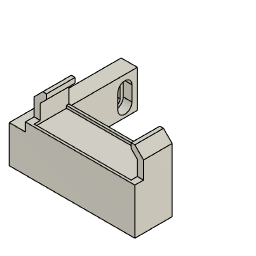
Nozzle brush (Autodesk Fusion 360 design; units mm, degrees)
Autodesk Fusion 360 part; units mm, degrees
sketch "Sketch1" plane through (0, 0, 0) normal (0, 1, 0) x (1, 0, 0)
  line L0 (0, 0) -> (6.5, 0)
  line L1 (6.5, 0) -> (6.5, -15)
  line L2 (6.5, -15) -> (0, -15)
  line L3 (0, -15) -> (0, 0)
  dimension "d1" = 6.5
  dimension "d2" = 15
  constraint horizontal L0
  constraint vertical L1
  constraint horizontal L2
  constraint vertical L3
  constraint coincident L0.start L3.end
  measures "d1" distance of L0.start L0.end
  measures "d2" distance of L0.start L2.end
extrude "Extrude1" add sketch "Sketch1" along normal blind 46.5
sketch "Sketch4" plane through (0, 0, 0) normal (0, -1, 0) x (1, 0, 0)
  line L0 (6.5, 15) -> (0, 15)
  line L1 (0, 15) -> (0, 0)
  line L2 (0, 0) -> (6.5, 0)
  line L3 (6.5, 0) -> (6.5, 15)
  line L4 (6.5, 15) -> (50.5, 15)
  line L5 (50.5, 15) -> (50.5, 29)
  line L6 (50.5, 29) -> (6.5, 29)
  line L7 (6.5, 29) -> (6.5, 15)
  line L8 (50.5, 15) -> (50.5, 0)
  line L9 (50.5, 0) -> (6.5, 0)
  dimension "d20" = 44
  dimension "d23" = 14
  dimension "d55" = 15
  constraint horizontal L4
  constraint vertical L5
  constraint horizontal L6
  constraint vertical L7
  constraint perpendicular L4 L8
  constraint coincident L2.end L3.start
  constraint horizontal L9
  constraint collinear L3 L7
  measures "d20" distance of L5.end L6.end
  measures "d23" distance of L4.end L5.end
  measures "d55" distance of L2 L4
extrude "Extrude5" add sketch "Sketch4" against normal blind 16.5
sketch "Sketch5" plane through (0, 16.5, 0) normal (0, 1, 0) x (-1, 0, 0)
  line L0 (-6.5, 15) -> (-6.5, 29)
  line L1 (-6.5, 29) -> (-50.5, 29)
  line L2 (-50.5, 29) -> (-50.5, 0)
  line L3 (-6.5, 0) -> (-6.5, 15)
  line L4 (-48, 27) -> (-9, 27)
  line L5 (-9, 27) -> (-9, 17.5)
  line L6 (-9, 17.5) -> (-48, 17.5)
  line L7 (-48, 17.5) -> (-48, 27)
  line L8 (-50.5, 0) -> (-6.5, 0)
  dimension "d25" = 2.5
  dimension "d26" = 2.5
  dimension "d27" = 2
  dimension "d60" = 9.5
  constraint horizontal L4
  constraint vertical L5
  constraint horizontal L6
  constraint vertical L7
  measures "d25" distance of L0 L5
  measures "d26" distance of L2 L7
  measures "d27" distance of L1 L4
  measures "d60" distance of L4.start L6.end
extrude "Extrude6" cut sketch "Sketch5" against normal up to surface (14 mm away) contours L4 L5 L6 L7
chamfer "Chamfer3" distance 2.5 angle 45 3 edges at (48, 9.5, 27) (28.5, 2.5, 27) (9, 9.5, 27)
extrude "Extrude7" cut 1 faces at (34.1667, 12.6667, 27) along direction (0, 0, 1) through all
chamfer "Chamfer4" distance 3.5 angle 45 3 edges at (50.5, 8.25, 29) (28.5, 0, 29) (6.5, 8.25, 29)
sketch "Sketch7" plane through (6.5, 0, 0) normal (1, 0, 0) x (0, 1, 0)
  line L0 (16.5, 0) -> (46.5, 0)
  line L1 (46.5, 0) -> (46.5, 15)
  line L2 (46.5, 15) -> (16.5, 15)
  line L3 (16.5, 15) -> (16.5, 0)
  line L4 (43.1, 4) -> (43.1, 10)
  arc A0 (43.1, 10) -> (39.9, 10) centre (41.5, 10) ccw
  line L5 (39.9, 10) -> (39.9, 4)
  arc A1 (39.9, 4) -> (43.1, 4) centre (41.5, 4) ccw
  line L6 (41.5, 4) -> (41.5, 10) construction
  line L7 (22.1, 4) -> (22.1, 10)
  arc A2 (22.1, 10) -> (18.9, 10) centre (20.5, 10) ccw
  line L8 (18.9, 10) -> (18.9, 4)
  arc A3 (18.9, 4) -> (22.1, 4) centre (20.5, 4) ccw
  line L9 (20.5, 4) -> (20.5, 10) construction
  line L10 (41.5, 7) -> (46.5, 7) construction
  line L11 (20.5, 7) -> (41.5, 7) construction
  point P0 (41.5, 7)
  point P1 (20.5, 7)
  dimension "d37" = 3.2
  dimension "d38" = 6
  dimension "d44" = 5
  dimension "d61" = 4
  dimension "d62" = 7
  constraint tangent L4 A0
  constraint tangent A0 L5
  constraint parallel L4 L5
  constraint tangent L5 A1
  constraint tangent L4 A1
  constraint midpoint L6 P0
  constraint tangent L7 A2
  constraint tangent A2 L8
  constraint parallel L7 L8
  constraint tangent L8 A3
  constraint tangent L7 A3
  constraint midpoint L9 P1
  constraint equal L6 L9
  constraint equal A0 A2
  constraint coincident P0 L10.start
  constraint coincident L1 L10.end
  constraint perpendicular L1 L10
  constraint horizontal L11
  constraint vertical L9
  constraint vertical L6
  constraint coincident P1 L11.start
  measures "d37" diameter of A0
  measures "d38" distance of A1.centre A0.centre
  measures "d44" distance of P0 L10.end
  measures "d61" distance of L3 L9
  measures "d62" distance of L0 L11
extrude "Extrude9" cut sketch "Sketch7" against normal through all contours L4 A0 L5 A1 | L7 A2 L8 A3
sketch "Sketch8" plane through (6.5, 0, 0) normal (1, 0, 0) x (0, 1, 0)
  line L0 (39.9, 4) -> (39.9, 10)
  arc A0 (43.1, 10) -> (39.9, 10) centre (41.5, 10) ccw
  line L1 (43.1, 10) -> (43.1, 4)
  arc A1 (39.9, 4) -> (43.1, 4) centre (41.5, 4) ccw
  line L2 (18.9, 4) -> (18.9, 10)
  arc A2 (22.1, 10) -> (18.9, 10) centre (20.5, 10) ccw
  line L3 (22.1, 10) -> (22.1, 4)
  arc A3 (18.9, 4) -> (22.1, 4) centre (20.5, 4) ccw
  line L4 (16.5, 0) -> (46.5, 0)
  line L5 (46.5, 0) -> (46.5, 15)
  line L6 (46.5, 15) -> (16.5, 15)
  line L7 (16.5, 15) -> (16.5, 0)
  line L8 (23.35, 4) -> (23.35, 10)
  arc A4 (23.35, 10) -> (17.65, 10) centre (20.5, 10) ccw
  line L9 (17.65, 10) -> (17.65, 4)
  arc A5 (17.65, 4) -> (23.35, 4) centre (20.5, 4) ccw
  line L10 (20.5, 4) -> (20.5, 10) construction
  line L11 (44.35, 4) -> (44.35, 10)
  arc A6 (44.35, 10) -> (38.65, 10) centre (41.5, 10) ccw
  line L12 (38.65, 10) -> (38.65, 4)
  arc A7 (38.65, 4) -> (44.35, 4) centre (41.5, 4) ccw
  line L13 (41.5, 4) -> (41.5, 10) construction
  point P0 (20.5, 7)
  point P1 (41.5, 7)
  dimension "d41" = 5.7
  constraint tangent L8 A4
  constraint tangent A4 L9
  constraint parallel L8 L9
  constraint tangent L9 A5
  constraint tangent L8 A5
  constraint parallel L3 L10
  constraint midpoint L10 P0
  constraint tangent L11 A6
  constraint tangent A6 L12
  constraint parallel L11 L12
  constraint tangent L12 A7
  constraint tangent L11 A7
  constraint midpoint L13 P1
  constraint equal A4 A6
  constraint equal L9 L12
  constraint concentric A2 A4
  constraint concentric A3 A5
  constraint concentric A0 A6
  constraint vertical L13
  measures "d41" distance of L8 L9
extrude "Extrude10" cut sketch "Sketch8" against normal blind 3.5 contours L8 A4 L9 A5 | L11 A6 L12 A7
sketch "Sketch9" plane through (0, 0, 17.5) normal (0, 0, 1) x (-1, 0, 0)
  line L0 (-9, -2.5) -> (-48, -2.5)
  line L1 (-48, -2.5) -> (-48, -16.5)
  line L2 (-48, -16.5) -> (-9, -16.5)
  line L3 (-9, -16.5) -> (-9, -2.5)
  line L4 (-9, -16.5) -> (-48, -16.5)
  line L5 (-48, -15.5) -> (-9, -15.5)
  dimension "d47" = 1
  constraint coincident L2.end L3.start
  constraint coincident L1.end L2.start
  constraint coincident L1 L5.start
  constraint coincident L3 L5.end
  constraint perpendicular L3 L5
  measures "d47" distance of L4 L5
extrude "Extrude11" add sketch "Sketch9" along normal blind 1 contours L1 L2 L3 L4 L5
ref_plane "WorkPlane1" through (50.5, 0, 25.5) normal (0, 0, -1) x (-1, 0, 0)
sketch "Sketch10" plane through (50.51, 0, 25.5) normal (0, 0, -1) x (1, 0, 0)
  line L0 (-44.01, -16.5) -> (-44.01, 0)
  line L1 (-5.01, -5) -> (-39.01, -5)
  line L2 (-5.01, -5) -> (-39.01, -5)
  line L3 (-5.01, -5) -> (0, -5)
  line L4 (0, -5) -> (0, 0)
  line L5 (0, 0) -> (-44.01, 0)
  line L6 (-44.01, 0) -> (-44.01, -5)
  line L7 (-44.01, -5) -> (-39.01, -5)
  constraint coincident L1.start L2.start
  constraint coincident L1.end L2.end
  constraint parallel L1 L3
  constraint coincident L4.end L5.start
  constraint vertical L4
  constraint coincident L0.end L5.end
  constraint coincident L0 L6.end
  constraint perpendicular L5 L6
  constraint horizontal L7
extrude "Extrude12" cut sketch "Sketch10" against normal through all
extrude "Extrude14" cut 1 faces at (22.3333, 1.1667, 25.5) along direction (0, 0, -1) up to surface (7 mm away)
extrude "Extrude15" cut 1 faces at (35.8333, 0, 11.1667) along direction (0, 1, 0) blind 1.5
